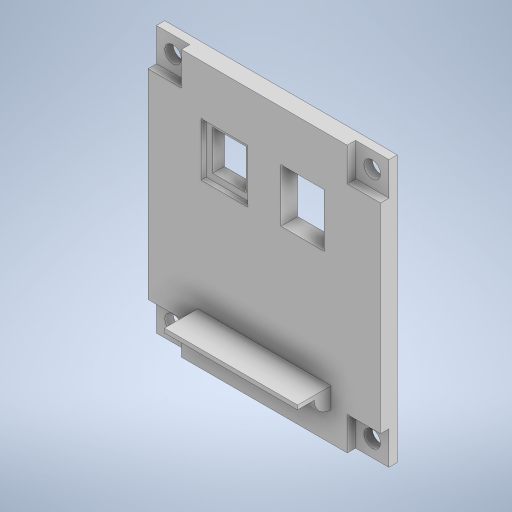
# Autodesk Inventor part: BackPannel
Saved by Autodesk Inventor 2023 (Build 270158000, 158)
## iProperties
Created: 2023-10-05
Part Number: BackPannel
Material: Generic
Document SubType Name: Modeling
Designer: Gage
Density: 1 g/cm^3
Appearance: Default
Author: Gage
## iProperties of the stored document BackPannel_3DPrint.ipt
Created: 2023-10-27
Part Number: BackPannel_3DPrint
Material: Generic
Document SubType Name: Modeling
Designer: Gage
Density: 1 g/cm^3
Appearance: Default
Author: Gage
Autodesk Inventor part; units mm, degrees
ref_plane "YZ Plane" through (0, 0, 0) normal (1, 0, 0) x (0, 1, 0)
ref_plane "XZ Plane" through (0, 0, 0) normal (0, 1, 0) x (-1, 0, 0)
ref_plane "XY Plane" through (0, 0, 0) normal (0, 0, 1) x (1, 0, 0)
sketch "Sketch1" plane through (0, 0, 0) normal (0, 0, 1) x (1, 0, 0)
  line L0 (-44.323, 50.8) -> (44.323, 50.8)
  line L1 (44.323, 50.8) -> (44.323, -50.8)
  line L2 (44.323, -50.8) -> (-44.323, -50.8)
  line L3 (-44.323, -50.8) -> (-44.323, 50.8)
  point P0 (0, 0)
  point P1 (0, 0)
  point P2 (0, 50.8)
  point P3 (44.323, 0)
  dimension "d0" = 88.646
  dimension "d1" = 101.6
  constraints: 8 end point, 2 midpoint, 2 parallel, 1 horizontal, 1 horizontal alignment, 1 perpendicular, 1 vertical alignment
  measures "d0" distance of L1.end L2.end
  measures "d1" distance of L0.end L1.end
extrude "Extrusion1" add sketch "Sketch1" along normal blind 6.35
sketch "Sketch2" plane through (0, 0, 6.35) normal (0, 0, 1) x (1, 0, 0)
  line L0 (-44.323, 50.8) -> (44.323, 50.8)
  line L1 (-44.323, 50.8) -> (-31.623, 50.8)
  line L2 (-31.623, 50.8) -> (-31.623, 38.1)
  line L3 (-31.623, 38.1) -> (-44.323, 38.1)
  line L4 (-44.323, 38.1) -> (-44.323, 50.8)
  line L5 (44.323, 50.8) -> (31.623, 50.8)
  line L6 (31.623, 50.8) -> (31.623, 38.1)
  line L7 (31.623, 38.1) -> (44.323, 38.1)
  line L8 (44.323, 38.1) -> (44.323, 50.8)
  line L9 (44.323, -50.8) -> (-44.323, -50.8)
  line L10 (44.323, -50.8) -> (31.623, -50.8)
  line L11 (31.623, -50.8) -> (31.623, -38.1)
  line L12 (31.623, -38.1) -> (44.323, -38.1)
  line L13 (44.323, -38.1) -> (44.323, -50.8)
  line L14 (-44.323, -50.8) -> (-31.623, -50.8)
  line L15 (-31.623, -50.8) -> (-31.623, -38.1)
  line L16 (-31.623, -38.1) -> (-44.323, -38.1)
  line L17 (-44.323, -38.1) -> (-44.323, -50.8)
  point P0 (0, 0)
  point P1 (0, 0)
  dimension "d4" = 12.7
  dimension "d5" = 12.7
  dimension "d6" = 12.7
  dimension "d7" = 12.7
  dimension "d8" = 12.7
  dimension "d9" = 12.7
  dimension "d10" = 12.7
  dimension "d11" = 12.7
  constraints: 36 end point, 8 parallel, 4 horizontal, 4 perpendicular
  measures "d4" distance of L3.start L3.end
  measures "d5" distance of L1.end L3.start
  measures "d6" distance of L7.end L7.start
  measures "d7" distance of L7.start L6.start
  measures "d8" distance of L12.start L12.end
  measures "d9" distance of L10.end L12.start
  measures "d10" distance of L16.end L16.start
  measures "d11" distance of L16.start L14.end
extrude "Extrusion2" cut sketch "Sketch2" against normal blind 3.175
sketch "Sketch3" plane through (0, 0, 3.175) normal (0, 0, 1) x (1, 0, 0)
  circle A0 centre (-37.973, 44.45) radius 3.175
  circle A1 centre (37.973, 44.45) radius 3.175
  circle A2 centre (37.973, -44.45) radius 3.175
  circle A3 centre (-37.973, -44.45) radius 3.175
  line L0 (-44.323, 50.8) -> (-31.623, 50.8)
  line L1 (-44.323, 38.1) -> (-44.323, 50.8)
  line L2 (31.623, 50.8) -> (44.323, 50.8)
  line L3 (44.323, 50.8) -> (44.323, 38.1)
  line L4 (44.323, -38.1) -> (44.323, -50.8)
  line L5 (44.323, -50.8) -> (31.623, -50.8)
  line L6 (-31.623, -50.8) -> (-44.323, -50.8)
  line L7 (-44.323, -50.8) -> (-44.323, -38.1)
  point P0 (0, 0)
  point P1 (0, 0)
  point P2 (-37.973, 50.8)
  point P3 (37.973, 50.8)
  point P4 (37.973, -50.8)
  point P5 (-37.973, -50.8)
  dimension "d14" = 6.35
  dimension "d15" = 6.35
  dimension "d16" = 6.35
  dimension "d17" = 6.35
  dimension "d18" = 6.35
  dimension "d19" = 6.35
  dimension "d20" = 6.35
  dimension "d21" = 6.35
  dimension "d22" = 6.35
  dimension "d23" = 6.35
  dimension "d24" = 6.35
  dimension "d25" = 6.35
  constraints: 16 end point, 4 centre point, 4 midpoint
  measures "d14" diameter of A0
  measures "d15" diameter of A1
  measures "d16" diameter of A2
  measures "d17" diameter of A3
  measures "d18" distance of point (-37.973, 50.8) A0.centre
  measures "d19" distance from line of L1 A0.centre
  measures "d20" distance of point (37.973, 50.8) A1.centre
  measures "d21" distance from line of L3 A1.centre
  measures "d22" distance from line of L4 A2.centre
  measures "d23" distance of point (37.973, -50.8) A2.centre
  measures "d24" distance of point (-37.973, -50.8) A3.centre
  measures "d25" distance from line of L7 A3.centre
extrude "Extrusion3" cut sketch "Sketch3" against normal blind 3.175
sketch "Sketch4" plane through (0, 0, 6.35) normal (0, 0, 1) x (1, 0, 0)
  line L0 (-25.4, -31.75) -> (25.4, -31.75)
  line L1 (25.4, -31.75) -> (25.4, -33.3502)
  line L2 (25.4, -33.3502) -> (-25.4, -33.3502)
  line L3 (-25.4, -33.3502) -> (-25.4, -31.75)
  line L4 (-31.623, -50.8) -> (31.623, -50.8) projected
  point P0 (0, 0)
  point P1 (0, -31.75)
  dimension "d28" = 50.8
  dimension "d29" = 1.6002
  dimension "d30" = 17.4498
  constraints: 8 end point, 2 parallel, 1 horizontal, 1 midpoint, 1 perpendicular, 1 vertical alignment
  measures "d28" distance of L1.end L2.end
  measures "d29" distance of L0.end L1.end
  measures "d30" distance between parallel lines of L4 L2
extrude "Extrusion4" add sketch "Sketch4" along normal blind 12.7
fillet "Fillet1" radius 6.35 1 edges at (0, -33.3502, 6.35) inverted yes
sketch "Sketch5" plane through (0, 0, 6.35) normal (0, 0, 1) x (1, 0, 0)
  line L0 (6.35, 31.75) -> (22.86, 31.75)
  line L1 (22.86, 31.75) -> (22.86, 11.43)
  line L2 (22.86, 11.43) -> (6.35, 11.43)
  line L3 (6.35, 11.43) -> (6.35, 31.75)
  line L4 (31.623, 50.8) -> (-31.623, 50.8) projected
  line L5 (-6.35, 31.75) -> (-24.13, 31.75)
  line L6 (-24.13, 31.75) -> (-24.13, 11.43)
  line L7 (-24.13, 11.43) -> (-6.35, 11.43)
  line L8 (-6.35, 11.43) -> (-6.35, 31.75)
  line L9 (-21.59, 29.21) -> (-8.89, 29.21)
  line L10 (-8.89, 29.21) -> (-8.89, 13.97)
  line L11 (-8.89, 13.97) -> (-21.59, 13.97)
  line L12 (-21.59, 13.97) -> (-21.59, 29.21)
  point P0 (0, 0)
  point P1 (14.605, 31.75)
  dimension "d34" = 16.51
  dimension "d35" = 20.32
  dimension "d36" = 19.05
  dimension "d44" = 6.35
  dimension "d45" = 17.78
  dimension "d46" = 20.32
  dimension "d47" = 19.05
  dimension "d48" = 6.35
  dimension "d49" = 12.7
  dimension "d50" = 15.24
  dimension "d51" = 2.54
  dimension "d52" = 2.54
  constraints: 24 end point, 6 parallel, 3 perpendicular, 2 horizontal, 1 midpoint
  measures "d34" distance of L1.end L2.end
  measures "d35" distance of L0.end L1.end
  measures "d36" distance between parallel lines of L0 L4
  measures "d44" distance from line of point (0, 0) L3
  measures "d45" distance of L7.end L6.end
  measures "d46" distance of L6.end L5.end
  measures "d47" distance between parallel lines of L4 L5
  measures "d48" distance from line of point (0, 0) L8
  measures "d49" distance of L10.end L11.end
  measures "d50" distance of L9.end L10.end
  measures "d51" distance between parallel lines of L6 L12
  measures "d52" distance between parallel lines of L7 L11
extrude "Extrusion5" cut sketch "Sketch5" against normal blind 25.4 contours L0 L1 L2 L3 | L9 L10 L11 L12
sketch "Sketch7" plane through (0, 0, 6.35) normal (0, 0, 1) x (1, 0, 0)
  line L0 (6.35, 31.75) -> (22.86, 31.75)
  line L1 (22.86, 31.75) -> (22.86, 11.43)
  line L2 (22.86, 11.43) -> (6.35, 11.43)
  line L3 (6.35, 11.43) -> (6.35, 31.75)
  line L4 (31.623, 50.8) -> (-31.623, 50.8)
  line L5 (-6.35, 31.75) -> (-24.13, 31.75)
  line L6 (-24.13, 31.75) -> (-24.13, 11.43)
  line L7 (-24.13, 11.43) -> (-6.35, 11.43)
  line L8 (-6.35, 11.43) -> (-6.35, 31.75)
  line L9 (-21.59, 29.21) -> (-8.89, 29.21)
  line L10 (-8.89, 29.21) -> (-8.89, 13.97)
  line L11 (-8.89, 13.97) -> (-21.59, 13.97)
  line L12 (-21.59, 13.97) -> (-21.59, 29.21)
  point P0 (0, 0)
  point P1 (0, 0)
  point P2 (14.605, 31.75)
  dimension "d53" = 16.51
  dimension "d54" = 20.32
  dimension "d55" = 19.05
  dimension "d56" = 6.35
  dimension "d57" = 17.78
  dimension "d58" = 20.32
  dimension "d59" = 19.05
  dimension "d60" = 6.35
  dimension "d61" = 12.7
  dimension "d62" = 15.24
  dimension "d63" = 2.54
  dimension "d64" = 2.54
  constraints: 26 end point, 6 parallel, 3 perpendicular, 2 horizontal, 1 midpoint
  measures "d53" distance of L2.start L2.end
  measures "d54" distance of L1.start L2.start
  measures "d55" distance between parallel lines of L0 L4
  measures "d56" distance from line of point (0, 0) L3
  measures "d57" distance of L7.end L7.start
  measures "d58" distance of L7.start L6.start
  measures "d59" distance between parallel lines of L4 L5
  measures "d60" distance from line of point (0, 0) L8
  measures "d61" distance of L11.start L11.end
  measures "d62" distance of L10.start L11.start
  measures "d63" distance between parallel lines of L6 L12
  measures "d64" distance between parallel lines of L7 L11
extrude "Extrusion7" cut sketch "Sketch7" against normal blind 1.905 contours L8 L7 L6 L5
body "Solid1"
